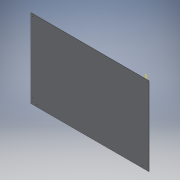
# Autodesk Inventor part: vrRig_enclosure_sidePanel
Saved by Autodesk Inventor 2016 (Build 200138000, 138)
## iProperties
Created: 2018-01-18
Part Number: vrRig_enclosure_sidePanel
Material: Generic
Document SubType Name: Modeling
Designer: harveylab
Density: 1 g/cm^3
Appearance: Default
Author: harveylab
Autodesk Inventor part; units mm, degrees
ref_plane "YZ Plane" through (0, 0, 0) normal (1, 0, 0) x (0, 1, 0)
ref_plane "XZ Plane" through (0, 0, 0) normal (0, 1, 0) x (-1, 0, 0)
ref_plane "XY Plane" through (0, 0, 0) normal (0, 0, 1) x (1, 0, 0)
ref_plane "Work Plane1" through (0, 0, 0) normal (0, 0, 1) x (1, 0, 0)
sketch "Sketch1" plane through (0, 0, 0) normal (0, 0, 1) x (1, 0, 0)
  line L0 (23.8808, -12.7) -> (23.8808, -25.4) projected
  line L1 (21.1808, -12.7) -> (23.8808, -12.7) projected
  line L2 (-728.3704, -532.9745) -> (-736.6, -532.9745) projected
  line L3 (-737.616, -531.9585) -> (-737.616, -523.7289) projected
  line L4 (-737.5192, -12.7) -> (-737.5192, -25.4) projected
  line L5 (-712.1334, -532.9746) -> (-0.9334, -532.9746) projected
  line L6 (23.8808, -25.4) -> (-738.1192, -25.4)
  line L7 (-738.1192, -25.4) -> (-738.1192, -533.4)
  line L8 (-738.1192, -533.4) -> (23.8808, -533.4)
  line L9 (23.8808, -533.4) -> (23.8808, -25.4)
  line L10 (23.8808, -25.4) -> (11.1808, -25.4)
  line L11 (11.1808, -25.4) -> (11.1808, -38.1)
  circle A0 centre (11.1808, -38.1) radius 3.302
  line L12 (23.8808, -533.4) -> (23.8808, -495.3)
  line L13 (23.8808, -495.3) -> (11.1808, -495.3)
  circle A1 centre (11.1808, -495.3) radius 3.302
  line L14 (23.8808, -533.4) -> (23.8808, -520.7)
  line L15 (23.8808, -520.7) -> (-14.2192, -520.7)
  circle A2 centre (-14.2192, -520.7) radius 3.302
  line L16 (23.8808, -533.4) -> (-357.1192, -533.4)
  line L17 (23.8808, -533.4) -> (404.8808, -533.4) construction
  line L18 (-357.1192, -533.4) -> (-357.1192, -428.4969)
  line L19 (-357.1192, -533.4) -> (-252.2161, -533.4) construction
  circle A3 centre (-725.4192, -38.1) radius 3.302
  circle A4 centre (-725.4192, -495.3) radius 3.302
  circle A5 centre (-700.0192, -520.7) radius 3.302
  point P0 (0, 0)
  dimension "d0" = 762
  dimension "d1" = 508
  dimension "d4" = 12.7
  dimension "d5" = 12.7
  dimension "d6" = 6.604
  dimension "d7" = 38.1
  dimension "d8" = 12.7
  dimension "d9" = 6.604
  dimension "d10" = 12.7
  dimension "d11" = 38.1
  dimension "d12" = 6.604
  dimension "d13" = 381
  dimension "d14" = 180
  dimension "d15" = 90
  constraints: 28 end point, 6 centre point, 4 perpendicular, 3 coincident, 3 horizontal, 3 point on line, 3 symmetric about line, 2 equal length, 2 parallel, 1 collinear, 3 other
  measures "d0" distance of L8.end L7.end
  measures "d1" distance of L7.end L6.end
  measures "d4" distance of L0.end L10.end
  measures "d5" distance of L10.end L11.end
  measures "d6" diameter of A0
  measures "d7" distance of L8.end L12.end
  measures "d8" distance of L12.end L13.end
  measures "d9" diameter of A1
  measures "d10" distance of L8.end L14.end
  measures "d11" distance of L14.end L15.end
  measures "d12" diameter of A2
  measures "d13" distance of L8.end L16.end
  measures "d14" angle of L16 L17
  measures "d15" angle of L19 L18
extrude "Extrusion2" add sketch "Sketch1" along normal blind 1.5875
body "Solid2"
